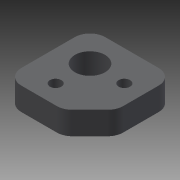
# Autodesk Inventor part: xShaftHolder
Saved by Autodesk Inventor 2013 (Build 170138000, 138)
## iProperties
Created: 2015-01-14
Part Number: xShaftHolder
Material: Generic
Document SubType Name: Modeling
Designer: dzban
Density: 1 g/cm^3
Author: dzban
Autodesk Inventor part; units mm, degrees
ref_plane "YZ Plane" through (0, 0, 0) normal (1, 0, 0) x (0, 1, 0)
ref_plane "XZ Plane" through (0, 0, 0) normal (0, 1, 0) x (-1, 0, 0)
ref_plane "XY Plane" through (0, 0, 0) normal (0, 0, 1) x (1, 0, 0)
sketch "Sketch1" plane through (0, 0, 0) normal (0, 0, 1) x (1, 0, 0)
  circle A0 centre (0, 0) radius 3.95
  circle A1 centre (0, -9) radius 1.5
  circle A2 centre (9, 0) radius 1.5
  line L0 (10, 8) -> (-4, 8)
  arc A3 (-4, 8) -> (-8, 4) centre (-4, 4) ccw
  line L1 (-8, 4) -> (-8, -10)
  arc A4 (-8, -10) -> (-4, -14) centre (-4, -10) ccw
  line L2 (-4, -14) -> (5.3431, -14)
  arc A5 (5.3431, -14) -> (8.1716, -12.8284) centre (5.3431, -10) ccw
  line L3 (8.1716, -12.8284) -> (12.8284, -8.1716)
  arc A6 (12.8284, -8.1716) -> (14, -5.3431) centre (10, -5.3431) ccw
  line L4 (14, -5.3431) -> (14, 4)
  arc A7 (14, 4) -> (10, 8) centre (10, 4) ccw
  constraints: 10 end point, 10 point on circle, 8 centre point
extrude "Extrusion1" add sketch "Sketch1" along normal blind 6
body "Solid1"
